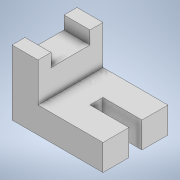
# Autodesk Inventor part: 7.1 Part 1
Saved by Autodesk Inventor 2020 (Build 240168000, 168)
## iProperties
Created: 2019-10-18
Part Number: 7.1 Part 1
Material: Generic
Document SubType Name: Modeling
Designer: cks4a449
Density: 1 g/cm^3
Appearance: Default
Author: cks4a449
Autodesk Inventor part; units mm, degrees
ref_plane "YZ Plane" through (0, 0, 0) normal (1, 0, 0) x (0, 1, 0)
ref_plane "XZ Plane" through (0, 0, 0) normal (0, 1, 0) x (-1, 0, 0)
ref_plane "XY Plane" through (0, 0, 0) normal (0, 0, 1) x (1, 0, 0)
sketch "Sketch1" plane through (0, 0, 0) normal (0, 0, 1) x (1, 0, 0)
  line L0 (0, 0) -> (9.2453, 0)
  line L1 (0, 0) -> (44.45, 0)
  line L2 (44.45, 0) -> (44.45, 12.7)
  line L3 (44.45, 12.7) -> (12.7, 12.7)
  line L4 (12.7, 12.7) -> (12.7, 31.75)
  line L5 (12.7, 31.75) -> (0, 31.75)
  line L6 (0, 31.75) -> (0, 0)
  dimension "d0" = 44.45
  dimension "d1" = 12.7
  dimension "d2" = 31.75
  dimension "d3" = 19.05
  dimension "d4" = 12.7
  constraints: 14 end point, 3 perpendicular, 2 horizontal, 1 point on line
  measures "d0" distance of L0.start L1.end
  measures "d1" distance of L1.end L2.end
  measures "d2" distance of L2.end L3.end
  measures "d3" distance of L3.end L4.end
  measures "d4" distance of L4.end L5.end
extrude "Extrusion1" add sketch "Sketch1" along normal blind 31.75
sketch "Sketch2" plane through (44.45, 0, 0) normal (1, 0, 0) x (0, 0, -1)
  line L0 (0, 12.7) -> (-31.75, 12.7) projected
  line L1 (-15.875, 12.7) -> (-12.7, 12.7)
  line L2 (-12.7, 12.7) -> (-19.05, 12.7)
  line L3 (-19.05, 12.7) -> (-19.05, 0)
  line L4 (-19.05, 0) -> (-12.7, 0)
  line L5 (-12.7, 0) -> (-12.7, 12.7)
  point P0 (0, 0)
  point P1 (-19.05, 12.7)
  dimension "d7" = 3.175
  dimension "d8" = 6.35
  dimension "d9" = 12.7
  constraints: 10 end point, 2 parallel, 1 horizontal, 1 midpoint, 1 perpendicular, 1 point on line
  measures "d7" distance of L1.start L1.end
  measures "d8" distance of L4.end L3.end
  measures "d9" distance of L3.end L2.end
extrude "Extrusion2" cut sketch "Sketch2" against normal blind 19.05
sketch "Sketch4" plane through (0, 31.75, 0) normal (0, 1, 0) x (1, 0, 0)
  line L0 (0, -25.4) -> (12.7, -25.4)
  line L1 (12.7, -25.4) -> (12.7, -6.35)
  line L2 (12.7, -6.35) -> (0, -6.35)
  line L3 (0, -6.35) -> (0, -25.4)
  line L4 (12.7, -31.75) -> (0, -31.75) projected
  line L5 (0, 0) -> (0, -31.75) projected
  dimension "d17" = 19.05
  dimension "d18" = 12.7
  dimension "d19" = 6.35
  dimension "d20" = 0
  constraints: 8 end point, 2 parallel, 1 horizontal, 1 perpendicular
  measures "d17" distance of L2.end L0.start
  measures "d18" distance of L1.end L2.end
  measures "d19" distance from line of L4 L0.start
  measures "d20" distance from line of L5 L0.start
extrude "Extrusion4" cut sketch "Sketch4" against normal blind 6.35
body "Solid1"
